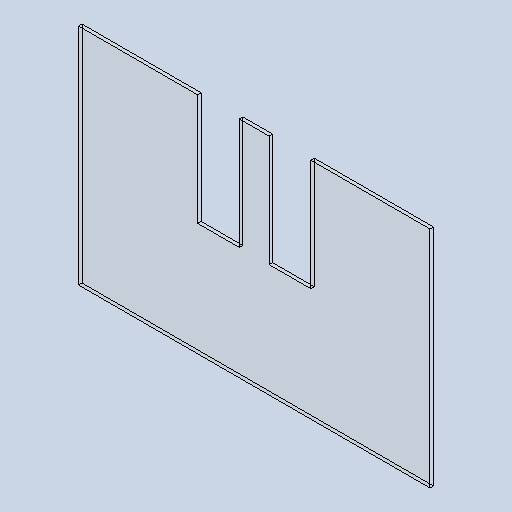
# Autodesk Inventor part: Toaster polycarb
Saved by Autodesk Inventor 2023.2 (Build 272271030, 271C)
## iProperties
Created: 2023-03-31
Part Number: Toaster polycarb
Material: Polycarbonate, Clear
Document SubType Name: Modeling
Designer: Main Account
Density: 1.2 g/cm^3
Appearance: Polycarbonate - Clear
Author: Main Account
Autodesk Inventor part; units mm, degrees
ref_plane "YZ Plane" through (0, 0, 0) normal (1, 0, 0) x (0, 1, 0)
ref_plane "XZ Plane" through (0, 0, 0) normal (0, 1, 0) x (-1, 0, 0)
ref_plane "XY Plane" through (0, 0, 0) normal (0, 0, 1) x (1, 0, 0)
sketch "Sketch1" plane through (0, 0, 0) normal (0, 0, 1) x (1, 0, 0)
  line L0 (-3.9687, 31.75) -> (-3.9687, -30.5843) construction
  line L1 (-2.8031, -31.75) -> (4.318, -31.75) construction
  line L2 (155.2031, -31.75) -> (148.082, -31.75) construction
  line L3 (156.3688, -30.5843) -> (156.3688, 31.75) construction
  line L4 (-6.35, 92.8585) -> (55.9843, 92.8585) construction
  line L5 (-3.9687, -31.75) -> (156.3688, -31.75)
  line L6 (156.3688, -31.75) -> (156.3688, 70.5878)
  line L7 (-3.9687, 70.5878) -> (-3.9687, -31.75)
  line L8 (102.0191, 70.5878) -> (82.9691, 70.5878)
  line L9 (82.9691, 70.5878) -> (82.9691, 19.7878)
  line L10 (82.9691, 19.7878) -> (102.0191, 19.7878)
  line L11 (102.0191, 19.7878) -> (102.0191, 70.5878)
  line L12 (50.3809, 70.5878) -> (69.4309, 70.5878)
  line L13 (69.4309, 70.5878) -> (69.4309, 19.7878)
  line L14 (69.4309, 19.7878) -> (50.3809, 19.7878)
  line L15 (50.3809, 19.7878) -> (50.3809, 70.5878)
  line L16 (156.3688, 70.5878) -> (69.4309, 70.5878)
  line L17 (50.3809, 70.5878) -> (-3.9687, 70.5878)
  point P0 (0, 0)
  dimension "d4" = 19.05
  dimension "d5" = 50.8
  dimension "d6" = 19.05
  dimension "d7" = 50.8
  constraints: 26 end point, 7 parallel, 3 horizontal, 3 perpendicular, 1 point on line
  measures "d4" distance of L10.end L9.end
  measures "d5" distance of L9.end L8.end
  measures "d6" distance of L13.end L14.end
  measures "d7" distance of L12.end L13.end
extrude "Extrusion1" add sketch "Sketch1" along normal blind 1.5875 contours L7 L17 L15 L14 L13 L16 L9 L10 L11 L6 L5
body "Solid1"
